Autodesk Inventor part; units mm, degrees
(part 6 of 6)
  spline S265 degree 5 poles (-92.4831, -154.5582) (-92.4852, -154.5654) (-92.5002, -154.6188) (-92.5281, -154.7186) (-92.5686, -154.8647) (-92.6211, -155.0575) (-92.6833, -155.29) (-92.7444, -155.5229) (-92.8044, -155.7563) (-92.8634, -155.9901) (-92.9213, -156.2244) (-92.9782, -156.4591) (-93.0341, -156.6942) (-93.089, -156.9297) (-93.1429, -157.1657) (-93.1958, -157.402) (-93.2478, -157.6387) (-93.2988, -157.8758) (-93.3488, -158.1133) (-93.3979, -158.3511) (-93.4461, -158.5893) (-93.4933, -158.8279) (-93.5397, -159.0668) (-93.5851, -159.306) (-93.6296, -159.5456) (-93.6732, -159.7855) (-93.716, -160.0258) (-93.7578, -160.2664) (-93.7988, -160.5073) (-93.8389, -160.7485) (-93.8782, -160.9901) (-93.9166, -161.2319) (-93.9541, -161.474) (-93.9908, -161.7165) (-94.0267, -161.9592) (-94.0617, -162.2022) (-94.096, -162.4455) (-94.1293, -162.6891) (-94.1619, -162.933) (-94.1937, -163.1771) (-94.2246, -163.4215) (-94.2548, -163.6662) (-94.2842, -163.9111) (-94.3184, -164.2054) (-94.346, -164.4509) (-94.3674, -164.6475) (-94.3832, -164.7951) (-94.3935, -164.8935) knots 0.383497 0.383497 0.383497 0.383497 0.383497 0.383497 0.385714 0.4 0.414286 0.428571 0.442857 0.457143 0.471429 0.485714 0.5 0.514286 0.528571 0.542857 0.557143 0.571429 0.585714 0.6 0.614286 0.628571 0.642857 0.657143 0.671429 0.685714 0.7 0.714286 0.728571 0.742857 0.757143 0.771429 0.785714 0.8 0.814286 0.828571 0.842857 0.857143 0.871429 0.885714 0.9 0.914286 0.928571 0.942857 0.957143 0.971429 1 1 1 1 1 1
  arc A133 (-94.3935, -164.8935) -> (-90.9204, -166.8337) centre (0, 0) ccw
  spline S266 degree 5 poles (-83.1213, -159.7881) (-83.1263, -159.7936) (-83.1639, -159.8344) (-83.2342, -159.9104) (-83.3374, -160.0215) (-83.4741, -160.1674) (-83.6394, -160.3422) (-83.8058, -160.5163) (-83.973, -160.6898) (-84.1412, -160.8626) (-84.3103, -161.0348) (-84.4803, -161.2063) (-84.6512, -161.3772) (-84.823, -161.5474) (-84.9956, -161.717) (-85.1691, -161.886) (-85.3434, -162.0543) (-85.5186, -162.2221) (-85.6946, -162.3892) (-85.8714, -162.5557) (-86.0489, -162.7216) (-86.2273, -162.8869) (-86.4065, -163.0516) (-86.5864, -163.2157) (-86.7671, -163.3793) (-86.9485, -163.5422) (-87.1307, -163.7046) (-87.3136, -163.8663) (-87.4973, -164.0275) (-87.6816, -164.1882) (-87.8667, -164.3482) (-88.0525, -164.5077) (-88.239, -164.6667) (-88.4262, -164.825) (-88.6141, -164.9829) (-88.8027, -165.1401) (-88.9919, -165.2968) (-89.1818, -165.453) (-89.3724, -165.6086) (-89.5636, -165.7636) (-89.7555, -165.9181) (-89.9481, -166.0721) (-90.1412, -166.2255) (-90.3738, -166.409) (-90.5684, -166.5612) (-90.7246, -166.6825) (-90.842, -166.7733) (-90.9204, -166.8337) knots 0.383497 0.383497 0.383497 0.383497 0.383497 0.383497 0.385714 0.4 0.414286 0.428571 0.442857 0.457143 0.471429 0.485714 0.5 0.514286 0.528571 0.542857 0.557143 0.571429 0.585714 0.6 0.614286 0.628571 0.642857 0.657143 0.671429 0.685714 0.7 0.714286 0.728571 0.742857 0.757143 0.771429 0.785714 0.8 0.814286 0.828571 0.842857 0.857143 0.871429 0.885714 0.9 0.914286 0.928571 0.942857 0.957143 0.971429 1 1 1 1 1 1
  spline S267 degree 3 poles (-81.233, -159.4491) (-81.5826, -159.271) (-82.3124, -159.1987) (-82.9219, -159.5716) (-83.1213, -159.7881) knots 0 0 0 0 0.571429 1 1 1 1
  arc A134 (-81.233, -159.4491) -> (-79.8928, -160.1248) centre (0, 0) ccw
  spline S268 degree 3 poles (-79.0425, -161.8446) (-78.987, -161.5556) (-79.0496, -160.8438) (-79.5417, -160.3) (-79.8928, -160.1248) knots 0 0 0 0 0.428571 1 1 1 1
  spline S269 degree 5 poles (-79.0425, -161.8446) (-79.0439, -161.8519) (-79.0544, -161.9064) (-79.0737, -162.0081) (-79.1016, -162.1572) (-79.1377, -162.3537) (-79.1799, -162.5907) (-79.221, -162.8279) (-79.261, -163.0656) (-79.2999, -163.3036) (-79.3378, -163.5419) (-79.3746, -163.7806) (-79.4104, -164.0196) (-79.4451, -164.2589) (-79.4788, -164.4985) (-79.5115, -164.7385) (-79.5432, -164.9788) (-79.5739, -165.2193) (-79.6036, -165.4602) (-79.6323, -165.7013) (-79.6601, -165.9428) (-79.687, -166.1845) (-79.7129, -166.4264) (-79.7378, -166.6687) (-79.7619, -166.9112) (-79.785, -167.154) (-79.8072, -167.397) (-79.8285, -167.6402) (-79.8489, -167.8838) (-79.8684, -168.1275) (-79.8871, -168.3715) (-79.9048, -168.6157) (-79.9217, -168.8602) (-79.9377, -169.1049) (-79.9529, -169.3498) (-79.9672, -169.5949) (-79.9806, -169.8402) (-79.9932, -170.0858) (-80.005, -170.3315) (-80.016, -170.5775) (-80.0261, -170.8236) (-80.0354, -171.07) (-80.0439, -171.3165) (-80.0531, -171.6126) (-80.0597, -171.8595) (-80.0644, -172.0573) (-80.0675, -172.2057) (-80.0695, -172.3046) knots 0.383497 0.383497 0.383497 0.383497 0.383497 0.383497 0.385714 0.4 0.414286 0.428571 0.442857 0.457143 0.471429 0.485714 0.5 0.514286 0.528571 0.542857 0.557143 0.571429 0.585714 0.6 0.614286 0.628571 0.642857 0.657143 0.671429 0.685714 0.7 0.714286 0.728571 0.742857 0.757143 0.771429 0.785714 0.8 0.814286 0.828571 0.842857 0.857143 0.871429 0.885714 0.9 0.914286 0.928571 0.942857 0.957143 0.971429 1 1 1 1 1 1
  arc A135 (-80.0695, -172.3046) -> (-76.4444, -173.9432) centre (0, 0) ccw
  spline S270 degree 5 poles (-69.2708, -166.2616) (-69.2754, -166.2675) (-69.3094, -166.3114) (-69.373, -166.3931) (-69.4664, -166.5126) (-69.5902, -166.6695) (-69.7401, -166.8577) (-69.8911, -167.0453) (-70.0431, -167.2323) (-70.196, -167.4188) (-70.3499, -167.6047) (-70.5047, -167.79) (-70.6605, -167.9747) (-70.8172, -168.1589) (-70.9749, -168.3426) (-71.1334, -168.5256) (-71.2928, -168.7082) (-71.4531, -168.8901) (-71.6143, -169.0716) (-71.7763, -169.2525) (-71.9392, -169.4328) (-72.1029, -169.6127) (-72.2674, -169.792) (-72.4328, -169.9708) (-72.599, -170.149) (-72.7659, -170.3268) (-72.9337, -170.504) (-73.1022, -170.6807) (-73.2715, -170.8569) (-73.4416, -171.0326) (-73.6125, -171.2078) (-73.7841, -171.3825) (-73.9564, -171.5567) (-74.1295, -171.7303) (-74.3033, -171.9035) (-74.4779, -172.0762) (-74.6532, -172.2484) (-74.8292, -172.4201) (-75.0059, -172.5913) (-75.1833, -172.762) (-75.3613, -172.9322) (-75.5401, -173.1019) (-75.7196, -173.2712) (-75.9358, -173.4737) (-76.1168, -173.6419) (-76.2621, -173.776) (-76.3714, -173.8764) (-76.4444, -173.9432) knots 0.383497 0.383497 0.383497 0.383497 0.383497 0.383497 0.385714 0.4 0.414286 0.428571 0.442857 0.457143 0.471429 0.485714 0.5 0.514286 0.528571 0.542857 0.557143 0.571429 0.585714 0.6 0.614286 0.628571 0.642857 0.657143 0.671429 0.685714 0.7 0.714286 0.728571 0.742857 0.757143 0.771429 0.785714 0.8 0.814286 0.828571 0.842857 0.857143 0.871429 0.885714 0.9 0.914286 0.928571 0.942857 0.957143 0.971429 1 1 1 1 1 1
  spline S271 degree 3 poles (-67.4181, -165.7637) (-67.7816, -165.6159) (-68.5149, -165.6058) (-69.0905, -166.0291) (-69.2708, -166.2616) knots 0 0 0 0 0.571429 1 1 1 1
  arc A136 (-67.4181, -165.7637) -> (-66.0255, -166.3233) centre (0, 0) ccw
  spline S272 degree 3 poles (-65.0324, -167.9648) (-65.0016, -167.6721) (-65.1243, -166.9682) (-65.6608, -166.4681) (-66.0255, -166.3233) knots 0 0 0 0 0.428571 1 1 1 1
  spline S273 degree 5 poles (-65.0324, -167.9648) (-65.0332, -167.9722) (-65.039, -168.0274) (-65.0496, -168.1304) (-65.0648, -168.2813) (-65.084, -168.4802) (-65.106, -168.7198) (-65.1268, -168.9598) (-65.1466, -169.1999) (-65.1652, -169.4404) (-65.1827, -169.681) (-65.1991, -169.922) (-65.2145, -170.1631) (-65.2288, -170.4046) (-65.242, -170.6462) (-65.2542, -170.8881) (-65.2654, -171.1302) (-65.2756, -171.3725) (-65.2848, -171.615) (-65.293, -171.8577) (-65.3002, -172.1006) (-65.3065, -172.3437) (-65.3118, -172.587) (-65.3161, -172.8305) (-65.3195, -173.0742) (-65.3219, -173.318) (-65.3234, -173.5621) (-65.324, -173.8063) (-65.3237, -174.0506) (-65.3225, -174.2952) (-65.3204, -174.5398) (-65.3173, -174.7847) (-65.3134, -175.0297) (-65.3086, -175.2749) (-65.303, -175.5202) (-65.2964, -175.7656) (-65.289, -176.0112) (-65.2808, -176.2569) (-65.2717, -176.5028) (-65.2617, -176.7488) (-65.2509, -176.9949) (-65.2393, -177.2411) (-65.2268, -177.4875) (-65.2109, -177.7833) (-65.1966, -178.03) (-65.1845, -178.2274) (-65.175, -178.3755) (-65.1686, -178.4742) knots 0.383497 0.383497 0.383497 0.383497 0.383497 0.383497 0.385714 0.4 0.414286 0.428571 0.442857 0.457143 0.471429 0.485714 0.5 0.514286 0.528571 0.542857 0.557143 0.571429 0.585714 0.6 0.614286 0.628571 0.642857 0.657143 0.671429 0.685714 0.7 0.714286 0.728571 0.742857 0.757143 0.771429 0.785714 0.8 0.814286 0.828571 0.842857 0.857143 0.871429 0.885714 0.9 0.914286 0.928571 0.942857 0.957143 0.971429 1 1 1 1 1 1
  arc A137 (-65.1686, -178.4742) -> (-61.4176, -179.7995) centre (0, 0) ccw
  spline S274 degree 5 poles (-54.9213, -171.5373) (-54.9254, -171.5435) (-54.9555, -171.5901) (-55.012, -171.6769) (-55.0949, -171.8039) (-55.2049, -171.9707) (-55.3384, -172.171) (-55.4729, -172.3707) (-55.6084, -172.57) (-55.745, -172.7687) (-55.8826, -172.967) (-56.0211, -173.1648) (-56.1607, -173.362) (-56.3012, -173.5589) (-56.4427, -173.7552) (-56.5852, -173.951) (-56.7285, -174.1464) (-56.8728, -174.3414) (-57.018, -174.5358) (-57.1641, -174.7298) (-57.3111, -174.9233) (-57.459, -175.1164) (-57.6077, -175.309) (-57.7573, -175.5012) (-57.9078, -175.6929) (-58.0591, -175.8842) (-58.2112, -176.075) (-58.3641, -176.2653) (-58.5179, -176.4553) (-58.6725, -176.6448) (-58.8278, -176.8338) (-58.984, -177.0224) (-59.141, -177.2106) (-59.2987, -177.3983) (-59.4572, -177.5856) (-59.6165, -177.7724) (-59.7765, -177.9589) (-59.9373, -178.1449) (-60.0989, -178.3304) (-60.2612, -178.5156) (-60.4242, -178.7003) (-60.5879, -178.8846) (-60.7524, -179.0684) (-60.9506, -179.2886) (-61.1167, -179.4715) (-61.2501, -179.6175) (-61.3505, -179.7268) (-61.4176, -179.7995) knots 0.383497 0.383497 0.383497 0.383497 0.383497 0.383497 0.385714 0.4 0.414286 0.428571 0.442857 0.457143 0.471429 0.485714 0.5 0.514286 0.528571 0.542857 0.557143 0.571429 0.585714 0.6 0.614286 0.628571 0.642857 0.657143 0.671429 0.685714 0.7 0.714286 0.728571 0.742857 0.757143 0.771429 0.785714 0.8 0.814286 0.828571 0.842857 0.857143 0.871429 0.885714 0.9 0.914286 0.928571 0.942857 0.957143 0.971429 1 1 1 1 1 1
  spline S275 degree 3 poles (-53.1175, -170.884) (-53.4922, -170.7676) (-54.2237, -170.8197) (-54.7614, -171.2902) (-54.9213, -171.5373) knots 0 0 0 0 0.571429 1 1 1 1
  arc A138 (-53.1175, -170.884) -> (-51.6824, -171.3235) centre (0, 0) ccw
  spline S276 degree 3 poles (-50.5537, -172.8748) (-50.5479, -172.5806) (-50.7298, -171.8896) (-51.3067, -171.4368) (-51.6824, -171.3235) knots 0 0 0 0 0.428571 1 1 1 1
  spline S277 degree 5 poles (-50.5537, -172.8748) (-50.5538, -172.8823) (-50.5549, -172.9378) (-50.5568, -173.0413) (-50.5591, -173.1929) (-50.5614, -173.3928) (-50.563, -173.6334) (-50.5634, -173.8742) (-50.5627, -174.1152) (-50.5609, -174.3563) (-50.5579, -174.5976) (-50.5538, -174.8391) (-50.5487, -175.0807) (-50.5425, -175.3225) (-50.5352, -175.5644) (-50.5268, -175.8064) (-50.5175, -176.0486) (-50.5071, -176.2908) (-50.4957, -176.5333) (-50.4832, -176.7758) (-50.4698, -177.0184) (-50.4554, -177.2612) (-50.4401, -177.5041) (-50.4237, -177.7471) (-50.4064, -177.9901) (-50.3882, -178.2333) (-50.369, -178.4766) (-50.3489, -178.72) (-50.3279, -178.9634) (-50.3059, -179.207) (-50.283, -179.4506) (-50.2593, -179.6943) (-50.2346, -179.9381) (-50.209, -180.182) (-50.1826, -180.4259) (-50.1552, -180.6699) (-50.127, -180.914) (-50.098, -181.1581) (-50.0681, -181.4024) (-50.0373, -181.6466) (-50.0056, -181.8909) (-49.9732, -182.1353) (-49.9399, -182.3797) (-49.8989, -182.6731) (-49.8637, -182.9177) (-49.8349, -183.1133) (-49.813, -183.2601) (-49.7981, -183.358) knots 0.383497 0.383497 0.383497 0.383497 0.383497 0.383497 0.385714 0.4 0.414286 0.428571 0.442857 0.457143 0.471429 0.485714 0.5 0.514286 0.528571 0.542857 0.557143 0.571429 0.585714 0.6 0.614286 0.628571 0.642857 0.657143 0.671429 0.685714 0.7 0.714286 0.728571 0.742857 0.757143 0.771429 0.785714 0.8 0.814286 0.828571 0.842857 0.857143 0.871429 0.885714 0.9 0.914286 0.928571 0.942857 0.957143 0.971429 1 1 1 1 1 1
  arc A139 (-49.7981, -183.358) -> (-45.9483, -184.3604) centre (0, 0) ccw
  spline S278 degree 5 poles (-40.1761, -175.577) (-40.1796, -175.5835) (-40.2057, -175.6325) (-40.2546, -175.7238) (-40.3265, -175.8573) (-40.4219, -176.0329) (-40.5379, -176.2437) (-40.655, -176.4542) (-40.7731, -176.6642) (-40.8924, -176.8738) (-41.0126, -177.083) (-41.1339, -177.2918) (-41.2563, -177.5003) (-41.3796, -177.7083) (-41.5039, -177.9159) (-41.6292, -178.1231) (-41.7555, -178.33) (-41.8828, -178.5364) (-42.011, -178.7425) (-42.1401, -178.9482) (-42.2701, -179.1535) (-42.4011, -179.3584) (-42.5329, -179.5629) (-42.6657, -179.7671) (-42.7994, -179.9709) (-42.9339, -180.1743) (-43.0693, -180.3773) (-43.2055, -180.58) (-43.3426, -180.7823) (-43.4806, -180.9842) (-43.6194, -181.1857) (-43.759, -181.3869) (-43.8994, -181.5877) (-44.0407, -181.7881) (-44.1827, -181.9882) (-44.3256, -182.1879) (-44.4692, -182.3872) (-44.6137, -182.5861) (-44.7589, -182.7847) (-44.9049, -182.983) (-45.0517, -183.1809) (-45.1992, -183.3784) (-45.3475, -183.5755) (-45.5263, -183.8117) (-45.6763, -184.008) (-45.7969, -184.1648) (-45.8876, -184.2822) (-45.9483, -184.3604) knots 0.383497 0.383497 0.383497 0.383497 0.383497 0.383497 0.385714 0.4 0.414286 0.428571 0.442857 0.457143 0.471429 0.485714 0.5 0.514286 0.528571 0.542857 0.557143 0.571429 0.585714 0.6 0.614286 0.628571 0.642857 0.657143 0.671429 0.685714 0.7 0.714286 0.728571 0.742857 0.757143 0.771429 0.785714 0.8 0.814286 0.828571 0.842857 0.857143 0.871429 0.885714 0.9 0.914286 0.928571 0.942857 0.957143 0.971429 1 1 1 1 1 1
  spline S279 degree 3 poles (-38.4341, -174.7731) (-38.8174, -174.6888) (-39.5419, -174.8028) (-40.0377, -175.3172) (-40.1761, -175.577) knots 0 0 0 0 0.571429 1 1 1 1
  arc A140 (-38.4341, -174.7731) -> (-36.967, -175.0893) centre (0, 0) ccw
  spline S280 degree 3 poles (-35.7108, -176.5393) (-35.7299, -176.2456) (-35.9698, -175.5726) (-36.583, -175.1703) (-36.967, -175.0893) knots 0 0 0 0 0.428571 1 1 1 1
  spline S281 degree 5 poles (-35.7108, -176.5393) (-35.7103, -176.5467) (-35.7067, -176.6021) (-35.6998, -176.7054) (-35.6892, -176.8567) (-35.6746, -177.056) (-35.6557, -177.2959) (-35.6357, -177.5359) (-35.6146, -177.776) (-35.5923, -178.0161) (-35.5688, -178.2563) (-35.5443, -178.4965) (-35.5187, -178.7368) (-35.492, -178.9772) (-35.4642, -179.2176) (-35.4354, -179.458) (-35.4055, -179.6985) (-35.3746, -179.9391) (-35.3427, -180.1796) (-35.3097, -180.4202) (-35.2758, -180.6609) (-35.2409, -180.9015) (-35.205, -181.1422) (-35.1681, -181.383) (-35.1302, -181.6237) (-35.0914, -181.8645) (-35.0517, -182.1052) (-35.011, -182.346) (-34.9694, -182.5868) (-34.9269, -182.8276) (-34.8834, -183.0684) (-34.8391, -183.3093) (-34.7938, -183.5501) (-34.7476, -183.7909) (-34.7006, -184.0317) (-34.6527, -184.2725) (-34.6039, -184.5133) (-34.5542, -184.7541) (-34.5037, -184.9949) (-34.4523, -185.2357) (-34.4001, -185.4764) (-34.347, -185.7172) (-34.2931, -185.9579) (-34.2274, -186.2468) (-34.1716, -186.4874) (-34.1263, -186.68) (-34.092, -186.8243) (-34.0689, -186.9206) knots 0.383497 0.383497 0.383497 0.383497 0.383497 0.383497 0.385714 0.4 0.414286 0.428571 0.442857 0.457143 0.471429 0.485714 0.5 0.514286 0.528571 0.542857 0.557143 0.571429 0.585714 0.6 0.614286 0.628571 0.642857 0.657143 0.671429 0.685714 0.7 0.714286 0.728571 0.742857 0.757143 0.771429 0.785714 0.8 0.814286 0.828571 0.842857 0.857143 0.871429 0.885714 0.9 0.914286 0.928571 0.942857 0.957143 0.971429 1 1 1 1 1 1
  arc A141 (-34.0689, -186.9206) -> (-30.1479, -187.5929) centre (0, 0) ccw
  spline S282 degree 5 poles (-25.1414, -178.3516) (-25.1443, -178.3585) (-25.1662, -178.4095) (-25.2071, -178.5046) (-25.2675, -178.6437) (-25.3477, -178.8267) (-25.4454, -179.0467) (-25.5442, -179.2663) (-25.6441, -179.4856) (-25.7451, -179.7045) (-25.8472, -179.9232) (-25.9503, -180.1416) (-26.0546, -180.3596) (-26.1598, -180.5773) (-26.2661, -180.7947) (-26.3734, -181.0119) (-26.4817, -181.2287) (-26.5909, -181.4452) (-26.7012, -181.6614) (-26.8124, -181.8773) (-26.9246, -182.0928) (-27.0377, -182.3081) (-27.1517, -182.5231) (-27.2667, -182.7378) (-27.3826, -182.9522) (-27.4994, -183.1663) (-27.617, -183.38) (-27.7356, -183.5935) (-27.8551, -183.8067) (-27.9754, -184.0196) (-28.0966, -184.2322) (-28.2187, -184.4444) (-28.3416, -184.6564) (-28.4653, -184.8681) (-28.5899, -185.0795) (-28.7153, -185.2906) (-28.8415, -185.5014) (-28.9686, -185.7119) (-29.0964, -185.9221) (-29.2251, -186.132) (-29.3545, -186.3416) (-29.4848, -186.5509) (-29.6158, -186.7599) (-29.774, -187.0104) (-29.9068, -187.2187) (-30.0136, -187.3852) (-30.0941, -187.5098) (-30.1479, -187.5929) knots 0.383497 0.383497 0.383497 0.383497 0.383497 0.383497 0.385714 0.4 0.414286 0.428571 0.442857 0.457143 0.471429 0.485714 0.5 0.514286 0.528571 0.542857 0.557143 0.571429 0.585714 0.6 0.614286 0.628571 0.642857 0.657143 0.671429 0.685714 0.7 0.714286 0.728571 0.742857 0.757143 0.771429 0.785714 0.8 0.814286 0.828571 0.842857 0.857143 0.871429 0.885714 0.9 0.914286 0.928571 0.942857 0.957143 0.971429 1 1 1 1 1 1
  spline S283 degree 3 poles (-23.4739, -177.4029) (-23.8629, -177.3514) (-24.5751, -177.5264) (-25.0255, -178.0811) (-25.1414, -178.3516) knots 0 0 0 0 0.571429 1 1 1 1
  arc A142 (-23.4739, -177.4029) -> (-21.9852, -177.5935) centre (0, 0) ccw
  spline S284 degree 3 poles (-20.6105, -178.9318) (-20.6545, -178.6408) (-20.9506, -177.9906) (-21.5958, -177.6418) (-21.9852, -177.5935) knots 0 0 0 0 0.428571 1 1 1 1
  spline S285 degree 5 poles (-20.6105, -178.9318) (-20.6094, -178.9392) (-20.6011, -178.994) (-20.5855, -179.0964) (-20.5622, -179.2463) (-20.5306, -179.4436) (-20.4915, -179.681) (-20.4512, -179.9185) (-20.4098, -180.1558) (-20.3672, -180.3932) (-20.3235, -180.6305) (-20.2787, -180.8678) (-20.2328, -181.1051) (-20.1858, -181.3423) (-20.1378, -181.5795) (-20.0886, -181.8167) (-20.0385, -182.0537) (-19.9873, -182.2908) (-19.9351, -182.5278) (-19.8818, -182.7647) (-19.8276, -183.0016) (-19.7724, -183.2385) (-19.7162, -183.4753) (-19.659, -183.712) (-19.6009, -183.9487) (-19.5418, -184.1853) (-19.4818, -184.4218) (-19.4209, -184.6583) (-19.359, -184.8947) (-19.2962, -185.131) (-19.2325, -185.3673) (-19.1678, -185.6034) (-19.1023, -185.8396) (-19.0359, -186.0756) (-18.9686, -186.3116) (-18.9004, -186.5474) (-18.8314, -186.7832) (-18.7615, -187.019) (-18.6907, -187.2546) (-18.6191, -187.4901) (-18.5466, -187.7256) (-18.4733, -187.961) (-18.3992, -188.1963) (-18.3092, -188.4785) (-18.2332, -188.7136) (-18.1718, -188.9016) (-18.1253, -189.0425) (-18.0942, -189.1365) knots 0.383497 0.383497 0.383497 0.383497 0.383497 0.383497 0.385714 0.4 0.414286 0.428571 0.442857 0.457143 0.471429 0.485714 0.5 0.514286 0.528571 0.542857 0.557143 0.571429 0.585714 0.6 0.614286 0.628571 0.642857 0.657143 0.671429 0.685714 0.7 0.714286 0.728571 0.742857 0.757143 0.771429 0.785714 0.8 0.814286 0.828571 0.842857 0.857143 0.871429 0.885714 0.9 0.914286 0.928571 0.942857 0.957143 0.971429 1 1 1 1 1 1
  arc A143 (-18.0942, -189.1365) -> (-14.1303, -189.4738) centre (0, 0) ccw
  spline S286 degree 5 poles (-9.9255, -179.8412) (-9.9279, -179.8483) (-9.9453, -179.901) (-9.9781, -179.9992) (-10.0264, -180.143) (-10.0908, -180.3322) (-10.1695, -180.5596) (-10.2493, -180.7868) (-10.3303, -181.0137) (-10.4123, -181.2405) (-10.4955, -181.467) (-10.5798, -181.6933) (-10.6651, -181.9194) (-10.7515, -182.1453) (-10.839, -182.3709) (-10.9275, -182.5964) (-11.017, -182.8216) (-11.1075, -183.0466) (-11.199, -183.2713) (-11.2915, -183.4959) (-11.385, -183.7202) (-11.4795, -183.9443) (-11.5749, -184.1682) (-11.6712, -184.3919) (-11.7685, -184.6153) (-11.8667, -184.8385) (-11.9658, -185.0615) (-12.0659, -185.2843) (-12.1668, -185.5068) (-12.2687, -185.7291) (-12.3714, -185.9512) (-12.475, -186.1731) (-12.5795, -186.3947) (-12.6848, -186.6161) (-12.791, -186.8373) (-12.8981, -187.0583) (-13.006, -187.279) (-13.1147, -187.4996) (-13.2243, -187.7198) (-13.3347, -187.9399) (-13.4459, -188.1597) (-13.5579, -188.3793) (-13.6708, -188.5987) (-13.8071, -188.8617) (-13.9218, -189.0805) (-14.0141, -189.2554) (-14.0837, -189.3865) (-14.1303, -189.4738) knots 0.383497 0.383497 0.383497 0.383497 0.383497 0.383497 0.385714 0.4 0.414286 0.428571 0.442857 0.457143 0.471429 0.485714 0.5 0.514286 0.528571 0.542857 0.557143 0.571429 0.585714 0.6 0.614286 0.628571 0.642857 0.657143 0.671429 0.685714 0.7 0.714286 0.728571 0.742857 0.757143 0.771429 0.785714 0.8 0.814286 0.828571 0.842857 0.857143 0.871429 0.885714 0.9 0.914286 0.928571 0.942857 0.957143 0.971429 1 1 1 1 1 1
  spline S287 degree 3 poles (-8.3445, -178.7545) (-8.7365, -178.7362) (-9.4313, -178.971) (-9.833, -179.5619) (-9.9255, -179.8412) knots 0 0 0 0 0.571429 1 1 1 1
  arc A144 (-8.3445, -178.7545) -> (-6.845, -178.8182) centre (0, 0) ccw
  spline S288 degree 3 poles (-5.3618, -180.0351) (-5.4303, -179.7489) (-5.7805, -179.1261) (-6.4529, -178.8332) (-6.845, -178.8182) knots 0 0 0 0 0.428571 1 1 1 1
  spline S289 degree 5 poles (-5.3618, -180.0351) (-5.3601, -180.0423) (-5.3472, -180.0963) (-5.3229, -180.197) (-5.2869, -180.3443) (-5.2388, -180.5383) (-5.1797, -180.7715) (-5.1194, -181.0047) (-5.058, -181.2377) (-4.9954, -181.4706) (-4.9318, -181.7034) (-4.867, -181.936) (-4.8011, -182.1685) (-4.7342, -182.4009) (-4.6662, -182.6332) (-4.5971, -182.8653) (-4.527, -183.0973) (-4.4559, -183.3291) (-4.3838, -183.5609) (-4.3107, -183.7924) (-4.2366, -184.0239) (-4.1615, -184.2552) (-4.0854, -184.4863) (-4.0084, -184.7174) (-3.9304, -184.9483) (-3.8514, -185.179) (-3.7716, -185.4096) (-3.6908, -185.64) (-3.6091, -185.8703) (-3.5264, -186.1005) (-3.4429, -186.3305) (-3.3585, -186.5603) (-3.2732, -186.7901) (-3.187, -187.0196) (-3.1, -187.249) (-3.012, -187.4783) (-2.9232, -187.7074) (-2.8336, -187.9363) (-2.7431, -188.1651) (-2.6518, -188.3937) (-2.5596, -188.6222) (-2.4666, -188.8505) (-2.3728, -189.0786) (-2.2592, -189.3522) (-2.1635, -189.58) (-2.0864, -189.7621) (-2.0281, -189.8986) (-1.9891, -189.9896) knots 0.383497 0.383497 0.383497 0.383497 0.383497 0.383497 0.385714 0.4 0.414286 0.428571 0.442857 0.457143 0.471429 0.485714 0.5 0.514286 0.528571 0.542857 0.557143 0.571429 0.585714 0.6 0.614286 0.628571 0.642857 0.657143 0.671429 0.685714 0.7 0.714286 0.728571 0.742857 0.757143 0.771429 0.785714 0.8 0.814286 0.828571 0.842857 0.857143 0.871429 0.885714 0.9 0.914286 0.928571 0.942857 0.957143 0.971429 1 1 1 1 1 1
  arc A145 (-1.9891, -189.9896) -> (1.9891, -189.9896) centre (0, 0) ccw
  spline S290 degree 5 poles (5.3618, -180.0351) (5.3601, -180.0423) (5.3472, -180.0963) (5.3229, -180.197) (5.2869, -180.3443) (5.2388, -180.5383) (5.1797, -180.7715) (5.1194, -181.0047) (5.058, -181.2377) (4.9954, -181.4706) (4.9318, -181.7034) (4.867, -181.936) (4.8011, -182.1685) (4.7342, -182.4009) (4.6662, -182.6332) (4.5971, -182.8653) (4.527, -183.0973) (4.4559, -183.3291) (4.3838, -183.5609) (4.3107, -183.7924) (4.2366, -184.0239) (4.1615, -184.2552) (4.0854, -184.4863) (4.0084, -184.7174) (3.9304, -184.9483) (3.8514, -185.179) (3.7716, -185.4096) (3.6908, -185.64) (3.6091, -185.8703) (3.5264, -186.1005) (3.4429, -186.3305) (3.3585, -186.5603) (3.2732, -186.7901) (3.187, -187.0196) (3.1, -187.249) (3.012, -187.4783) (2.9232, -187.7074) (2.8336, -187.9363) (2.7431, -188.1651) (2.6518, -188.3937) (2.5596, -188.6222) (2.4666, -188.8505) (2.3728, -189.0786) (2.2592, -189.3522) (2.1635, -189.58) (2.0864, -189.7621) (2.0281, -189.8986) (1.9891, -189.9896) knots 0.383497 0.383497 0.383497 0.383497 0.383497 0.383497 0.385714 0.4 0.414286 0.428571 0.442857 0.457143 0.471429 0.485714 0.5 0.514286 0.528571 0.542857 0.557143 0.571429 0.585714 0.6 0.614286 0.628571 0.642857 0.657143 0.671429 0.685714 0.7 0.714286 0.728571 0.742857 0.757143 0.771429 0.785714 0.8 0.814286 0.828571 0.842857 0.857143 0.871429 0.885714 0.9 0.914286 0.928571 0.942857 0.957143 0.971429 1 1 1 1 1 1
  spline S291 degree 3 poles (6.845, -178.8182) (6.4529, -178.8332) (5.7805, -179.1261) (5.4303, -179.7489) (5.3618, -180.0351) knots 0 0 0 0 0.571429 1 1 1 1
  arc A146 (6.845, -178.8182) -> (8.3445, -178.7545) centre (0, 0) ccw
  spline S292 degree 3 poles (9.9255, -179.8412) (9.833, -179.5619) (9.4313, -178.971) (8.7365, -178.7362) (8.3445, -178.7545) knots 0 0 0 0 0.428571 1 1 1 1
  spline S293 degree 5 poles (9.9255, -179.8412) (9.9279, -179.8483) (9.9453, -179.901) (9.9781, -179.9992) (10.0264, -180.143) (10.0908, -180.3322) (10.1695, -180.5596) (10.2493, -180.7868) (10.3303, -181.0137) (10.4123, -181.2405) (10.4955, -181.467) (10.5798, -181.6933) (10.6651, -181.9194) (10.7515, -182.1453) (10.839, -182.3709) (10.9275, -182.5964) (11.017, -182.8216) (11.1075, -183.0466) (11.199, -183.2713) (11.2915, -183.4959) (11.385, -183.7202) (11.4795, -183.9443) (11.5749, -184.1682) (11.6712, -184.3919) (11.7685, -184.6153) (11.8667, -184.8385) (11.9658, -185.0615) (12.0659, -185.2843) (12.1668, -185.5068) (12.2687, -185.7291) (12.3714, -185.9512) (12.475, -186.1731) (12.5795, -186.3947) (12.6848, -186.6161) (12.791, -186.8373) (12.8981, -187.0583) (13.006, -187.279) (13.1147, -187.4996) (13.2243, -187.7198) (13.3347, -187.9399) (13.4459, -188.1597) (13.5579, -188.3793) (13.6708, -188.5987) (13.8071, -188.8617) (13.9218, -189.0805) (14.0141, -189.2554) (14.0837, -189.3865) (14.1303, -189.4738) knots 0.383497 0.383497 0.383497 0.383497 0.383497 0.383497 0.385714 0.4 0.414286 0.428571 0.442857 0.457143 0.471429 0.485714 0.5 0.514286 0.528571 0.542857 0.557143 0.571429 0.585714 0.6 0.614286 0.628571 0.642857 0.657143 0.671429 0.685714 0.7 0.714286 0.728571 0.742857 0.757143 0.771429 0.785714 0.8 0.814286 0.828571 0.842857 0.857143 0.871429 0.885714 0.9 0.914286 0.928571 0.942857 0.957143 0.971429 1 1 1 1 1 1
  arc A147 (14.1303, -189.4738) -> (18.0942, -189.1365) centre (0, 0) ccw
  spline S294 degree 5 poles (20.6105, -178.9318) (20.6094, -178.9392) (20.6011, -178.994) (20.5855, -179.0964) (20.5622, -179.2463) (20.5306, -179.4436) (20.4915, -179.681) (20.4512, -179.9185) (20.4098, -180.1558) (20.3672, -180.3932) (20.3235, -180.6305) (20.2787, -180.8678) (20.2328, -181.1051) (20.1858, -181.3423) (20.1378, -181.5795) (20.0886, -181.8167) (20.0385, -182.0537) (19.9873, -182.2908) (19.9351, -182.5278) (19.8818, -182.7647) (19.8276, -183.0016) (19.7724, -183.2385) (19.7162, -183.4753) (19.659, -183.712) (19.6009, -183.9487) (19.5418, -184.1853) (19.4818, -184.4218) (19.4209, -184.6583) (19.359, -184.8947) (19.2962, -185.131) (19.2325, -185.3673) (19.1678, -185.6034) (19.1023, -185.8396) (19.0359, -186.0756) (18.9686, -186.3116) (18.9004, -186.5474) (18.8314, -186.7832) (18.7615, -187.019) (18.6907, -187.2546) (18.6191, -187.4901) (18.5466, -187.7256) (18.4733, -187.961) (18.3992, -188.1963) (18.3092, -188.4785) (18.2332, -188.7136) (18.1718, -188.9016) (18.1253, -189.0425) (18.0942, -189.1365) knots 0.383497 0.383497 0.383497 0.383497 0.383497 0.383497 0.385714 0.4 0.414286 0.428571 0.442857 0.457143 0.471429 0.485714 0.5 0.514286 0.528571 0.542857 0.557143 0.571429 0.585714 0.6 0.614286 0.628571 0.642857 0.657143 0.671429 0.685714 0.7 0.714286 0.728571 0.742857 0.757143 0.771429 0.785714 0.8 0.814286 0.828571 0.842857 0.857143 0.871429 0.885714 0.9 0.914286 0.928571 0.942857 0.957143 0.971429 1 1 1 1 1 1
  spline S295 degree 3 poles (21.9852, -177.5935) (21.5958, -177.6418) (20.9506, -177.9906) (20.6545, -178.6408) (20.6105, -178.9318) knots 0 0 0 0 0.571429 1 1 1 1
  circle A148 centre (0, 0) radius 5
  line L0 (-94.4626, -151.9857) -> (-92.3779, -148.6315)
  arc A149 (-129.2323, -118) -> (-63.1453, 163.2105) centre (0, 0) ccw
  line L1 (-92.3779, -148.6315) -> (-92.3779, 151.9006) construction
  line L2 (-63.1453, 163.2105) -> (-176.8042, 119.2365)
  line L3 (-92.3779, 151.9006) -> (-93.1845, 152.7726)
  constraints: 6 end point, 1 line through centre, 1 point on circle, 1 point on line, 1 vertical
extrude "Extrusion10" add sketch "Sketch12" against normal up to surface (5 mm away) contours S295 S294 A147 S293 S292 A146 S291 S290 A145 S289 S288 A144 S287 S286 A143 S285 S284 A142 S283 S282 A141 S281 S280 A140 S279 S278 A139 S277 S276 A138 S275 S274 A137 S273 S272 A136 S271 S270 A135 S269 S268 A134 S267 S266 A133 S265 S264 A132 L0 A149 L2 L3 S167 S166 A83 S165 S164 A82 S163 S162 A81 S161 S160 A80 S159 S158 A79 S157 S156 A78 S155 S154 A77 S153 S152 A76 S151 S150 A75 S149 S148 A74 S147 S146 A73 S145 S144 A72 S143 S142 A71 S141 S140 A70 S139 S138 A69 S137 S136 A68 S135 S134 A67 S133 S132 A66 S131 S130 A65 S129 S128 A64 S127 S126 A63 S125 S124 A62 S123 S122 A61 S121 S120 A60 S119 S118 A59 S117 S116 A58 S115 S114 A57 S113 S112 A56 S111 S110 A55 S109 S108 A54 S107 S106 A53 S105 S104 A52 S103 S102 A51 S101 S100 A50 S99 S98 A49 S97 S96 A48 S95 S94 A47 S93 S92 A46 S91 S90 A45 S89 S88 A44 S87 S86 A43 S85 S84 A42 S83 S82 A41 S81 S80 A40 S79 S78 A39 S77 S76 A38 S75 S74 A37 S73 S72 A36 S71 S70 A35 S69 S68 A34 S67 S66 A33 S65 S64 A32 S63 S62 A31 S61 S60 A30 S59 S58 A29 S57 S56 A28 S55 S54 A27 S53 S52 A26 S51 S50 A25 S49 S48 A24 S47 S46 A23 S45 S44 A22 S43 S42 A21 S41 S40 A20 S39 S38 A19 S37 S36 A18 S35 S34 A17 S33 S32 A16 S31 S30 A15 S29 S28 A14 S27 S26 A13 S25 S24 A12 S23 S22 A11 S21 S20 A10 S19 S18 A9 S17 S16 A8 S15 S14 A7 S13 S12 A6 S11 S10 A5 S9 S8 A4 S7 S6 A3 S5 S4 A2 S3 S2 A1 S1 S0 A0
sketch "Sketch13" plane through (0, 5, 0) normal (0, 1, 0) x (1, 0, 0)
  line L0 (-93.1845, 152.7726) -> (-92.3779, 151.9006) projected
  line L1 (-93.1845, 152.7726) -> (-108.6373, 160.1725)
  line L2 (-108.6373, 160.1725) -> (-115.0928, 143.1123)
  line L3 (-176.8042, 119.2365) -> (-92.3779, 151.9006) projected
  line L4 (-92.3779, -148.6315) -> (-94.4626, -151.9857) projected
  line L5 (-94.4626, -151.9857) -> (-103.0634, -156.5694)
  line L6 (-103.0634, -156.5694) -> (-108.6373, -137.1967)
  arc A0 (-129.2323, -118) -> (-92.3779, -148.6315) centre (0, 0) ccw projected
  constraints: 8 end point, 1 point on circle, 1 point on line
extrude "Extrusion11" add sketch "Sketch13" against normal up to surface (5 mm away)
fillet "Fillet5" radius 1 2 edges at (-94.4626, 2.5, 151.9857) (-93.1845, 2.5, -152.7726)
fillet "Fillet6" radius 5 2 edges at (-108.6373, 2.5, -160.1725) (-103.0634, 2.5, 156.5694)
fillet "Fillet7" radius 30 3 edges at (-115.0928, 2.5, -143.1123) (-108.6373, 2.5, 137.1967) (-129.2323, 2.5, 118)
sketch "Sketch14" plane through (0, 5, 0) normal (0, 1, 0) x (1, 0, 0)
  arc A0 (99.92, 140) -> (-99.92, 140) centre (0, 0) ccw
  line L0 (99.92, 140) -> (-99.92, 140)
  line L1 (125.2, 105.3) -> (125.2, 85.3) projected
  line L2 (125.2, 105.3) -> (137.7717, 88.7957) construction
  line L3 (137.7717, 88.7957) -> (153.4787, 60.9572) construction
  line L4 (153.4787, 60.9572) -> (163.4393, 20.9872) construction
  line L5 (163.4393, 20.9872) -> (154.3726, 14.3468) construction
  line L6 (154.3726, 14.3468) -> (142.3688, 9.4942) construction
  line L7 (142.3688, 9.4942) -> (142.3688, 0) construction
  spline S0 degree 4 poles (125.2, 105.3) (137.7717, 88.7957) (153.4787, 60.9572) (163.4393, 20.9872) (154.3726, 14.3468) (142.3688, 9.4942) (142.3688, 0) knots 1 1 1 1 1 2 3 4 4 4 4 4
  arc A1 (120.2, 80.3) -> (125.2, 85.3) centre (120.2, 85.3) ccw projected
  line L8 (120.2, 80.3) -> (105.2, 80.3) projected
  arc A2 (105.2, 80.3) -> (100.2, 75.3) centre (105.2, 75.3) ccw projected
  line L9 (100.2, 75.3) -> (100.2, -75.3) projected
  line L10 (100.2, 0) -> (142.3688, 0)
  dimension "d107" = 140
  dimension "d108" = 172
  constraints: 4 end point, 2 horizontal, 2 point on circle, 1 centre point, 1 coincident, 1 midpoint, 1 parallel, 3 other
  measures "d107" distance from line of point (0, 0) L0
  measures "d108" radius of A0
extrude "Extrusion12" cut sketch "Sketch14" against normal through all
fillet "Fillet8" radius 5 2 edges at (-99.92, 2.5, -140) (99.92, 2.5, -140)
mirror "Mirror2" about plane through (0, 0, 0) normal (0, 0, 1) of "Extrusion12", "Fillet8"
body "Solid1"
